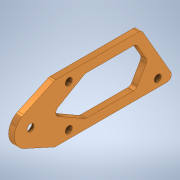
# Autodesk Inventor part: frame_side
Saved by Autodesk Inventor 2021 (Build 250183000, 183)
## iProperties
Created: 2022-05-14
Part Number: frame_side
Material: Generic
Document SubType Name: Modeling
Designer: ermoz
Density: 1 g/cm^3
Appearance: Default
Author: ermoz
Autodesk Inventor part; units mm, degrees
ref_plane "YZ Plane" through (0, 0, 0) normal (1, 0, 0) x (0, 1, 0)
ref_plane "XZ Plane" through (0, 0, 0) normal (0, 1, 0) x (-1, 0, 0)
ref_plane "XY Plane" through (0, 0, 0) normal (0, 0, 1) x (1, 0, 0)
sketch "Sketch1" plane through (0, 0, 0) normal (1, 0, 0) x (0, 1, 0)
  line L0 (0, 0) -> (50, 0)
  line L1 (50, 0) -> (50, 110)
  line L2 (50, 110) -> (0, 110)
  line L3 (0, 110) -> (0, 0)
  line L4 (50, 0) -> (0, -28.8675)
  line L5 (0, -28.8675) -> (0, 0)
  dimension "d0" = 110
  dimension "d1" = 50
  dimension "d68" = 60
  constraints: 12 end point, 2 parallel, 1 horizontal, 1 perpendicular, 1 vertical
  measures "d0" distance between parallel lines of L0 L2
  measures "d1" distance between parallel lines of L3 L1
  measures "d68" angle of L5 L4
extrude "Extrusion1" add sketch "Sketch1" along normal blind 5
fillet "Fillet1" radius 4 2 edges at (2.5, 50, 0) (2.5, 0, -28.8675)
sketch "Sketch2" plane through (5, 0, 0) normal (1, 0, 0) x (0, 0, -1)
  line L0 (-2.3094, 50) -> (-110, 50) projected
  line L1 (-110, 50) -> (-110, 0) projected
  line L2 (-110, 33.9915) -> (-75, 50)
  line L3 (-110, 16.0085) -> (-75, 0)
  line L4 (-110, 50) -> (-56.045, 50)
  line L5 (-56.045, 50) -> (-56.045, 0)
  line L6 (-56.045, 0) -> (-110, 0)
  line L7 (-110, 0) -> (-110, 50)
  line L8 (-110, 33.9915) -> (-110, 16.0085)
  line L9 (-110, 50) -> (-110, 0) projected
  line L10 (-110, 0) -> (-75, 0)
  circle A0 centre (-96, 25) radius 14
  circle A1 centre (-96, 25) radius 8.05
  line L11 (-96, 25) -> (-90.3078, 19.3078)
  line L12 (-96, 25) -> (-87.95, 25) construction
  circle A2 centre (-90.3078, 19.3078) radius 1.5
  circle A3 centre (-90.3078, 30.6922) radius 1.5
  circle A4 centre (-101.6922, 30.6922) radius 1.5
  circle A5 centre (-101.6922, 19.3078) radius 1.5
  circle A6 centre (-96, 25) radius 3
  point P0 (0, 0)
  point P1 (-110, 0)
  point P2 (-75, 0)
  point P3 (-110, 25)
  point P4 (-101.8232, 37.7315)
  point P5 (-101.8232, 12.2685)
  dimension "d84" = 16.1
  dimension "d13" = 35
  dimension "d82" = 28
  dimension "d83" = 25
  dimension "d86" = 45
  dimension "d87" = 3
  dimension "d90" = 360
  dimension "d97" = 6
  constraints: 20 end point, 6 centre point, 3 coincident, 2 equal length, 2 horizontal, 2 parallel, 2 perpendicular, 2 tangent, 1 collinear, 1 point on line, 1 vertical, 1 vertical alignment, 12 other
  measures "d13" distance from line of L1 L2.end
  measures "d82" diameter of A0
  measures "d83" distance from line of L0 A0.centre
  measures "d86" angle of L11 L12
  measures "d87" diameter of A2
  measures "d97" diameter of A6
extrude "Extrusion2" cut sketch "Sketch2" against normal blind 5 contours L2 L1 L0 | A0 L1 L2 | L6 L1 L3 | A0 L3 L1 | A6
fillet "Fillet3" radius 4 1 edges at (2.5, 50, 75)
chamfer "Chamfer2" distance 4 angle 45 1 edges at (0, 25, 99)
sketch "Sketch7" plane through (0, 0, 0) normal (-1, 0, 0) x (0, 0, 1)
  circle A0 centre (63, 43) radius 3
  circle A1 centre (63, 7) radius 3
  circle A2 centre (-14, 7) radius 3
  line L0 (74.1286, 0) -> (-21.9393, 0) projected
  line L1 (2.3094, 50) -> (74.1286, 50) projected
  point P0 (0, 0)
  dimension "d101" = 14
  dimension "d102" = 63
  dimension "d103" = 7
  dimension "d104" = 7
  dimension "d105" = 6
  constraints: 3 centre point, 2 equal radius, 1 horizontal alignment, 1 vertical alignment
  measures "d101" horizontal distance of A2.centre point (0, 0)
  measures "d102" horizontal distance of A1.centre point (0, 0)
  measures "d103" distance from line of L0 A1.centre
  measures "d104" distance from line of L1 A0.centre
  measures "d105" diameter of A0
extrude "Extrusion7" cut sketch "Sketch7" against normal blind 7
sketch "Sketch8" plane through (0, 0, 0) normal (-1, 0, 0) x (0, 0, 1)
  line L0 (4.6188, 42) -> (48.7321, 42)
  line L1 (48.7321, 42) -> (48.7321, 8)
  line L2 (48.7321, 8) -> (4.6188, 8)
  line L3 (4.6188, 8) -> (4.6188, 42)
  line L4 (4.6188, 42) -> (-5.1962, 25)
  line L5 (-5.1962, 25) -> (4.6188, 8)
  line L6 (48.7321, 8) -> (78.1769, 25)
  line L7 (78.1769, 25) -> (48.7321, 42)
  line L8 (-25.4034, 6) -> (-1.1547, 48) projected
  line L9 (2.3094, 50) -> (74.1286, 50) projected
  line L10 (74.1286, 0) -> (-21.9393, 0) projected
  circle A0 centre (63, 43) radius 3 projected
  point P0 (0, 0)
  dimension "d108" = 8
  dimension "d109" = 8
  dimension "d110" = 8
  dimension "d111" = 8
  constraints: 16 end point, 3 equal length, 3 parallel, 1 horizontal, 1 perpendicular
  measures "d108" distance between parallel lines of L9 L0
  measures "d109" distance between parallel lines of L10 L2
  measures "d110" distance between parallel lines of L8 L4
  measures "d111" distance from line of A0.centre L7
extrude "Extrusion8" cut sketch "Sketch8" against normal blind 7 contours L0 L1 L2 L3 | L3 L5 L4 | L7 L6 L1
fillet "Fillet5" radius 4 6 edges at (2.5, 42, 4.6188) (2.5, 25, -5.1962) (2.5, 8, 4.6188) (2.5, 8, 48.7321) (2.5, 25, 78.1769) (2.5, 42, 48.7321)
body "Solid1"
